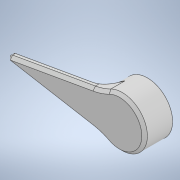
# Autodesk Inventor part: Стрелочка
Saved by Autodesk Inventor 2021.2 (Build 252289000, 289)
## iProperties
Created: 2024-11-30
Part Number: Стрелочка
Material: Типовые
Document SubType Name: Modeling
Designer: Barcock
Density: 1 g/cm^3
Appearance: По умолчанию
Author: Barcock
Autodesk Inventor part; units mm, degrees
ref_plane "YZ Plane" through (0, 0, 0) normal (1, 0, 0) x (0, 1, 0)
ref_plane "XZ Plane" through (0, 0, 0) normal (0, 1, 0) x (-1, 0, 0)
ref_plane "XY Plane" through (0, 0, 0) normal (0, 0, 1) x (1, 0, 0)
sketch "Эскиз1" plane through (0, 0, 0) normal (0, 0, 1) x (1, 0, 0)
  circle A0 centre (0, 0) radius 3.3
  circle A1 centre (0, 0) radius 4.5
  circle A2 centre (0, 0) radius 20 construction
  arc A3 (-19.586824, 0.492404) -> (-19.586824, -0.492404) centre (-19.5, 0) ccw
  line L0 (-19.586824, 0.492404) -> (-4.785745, 3.102233)
  arc A4 (-4.785745, 3.102233) -> (-2.024139, 4.019062) centre (-6.522227, 12.950311) ccw
  line L1 (-19.586824, -0.492404) -> (-4.785745, -3.102233)
  arc A5 (-2.024139, -4.019062) -> (-4.785745, -3.102233) centre (-6.522227, -12.950311) ccw
  dimension "d0" = 6.6
  dimension "d1" = 1.2
  dimension "d2" = 40
  dimension "d3" = 0.5
  dimension "d4" = 20
  dimension "d5" = 10
  constraints: 8 point on circle, 7 tangent, 6 centre point, 4 end point, 3 coincident, 1 equal length, 1 equal radius, 1 horizontal alignment
  measures "d0" diameter of A0
  measures "d1" radial gap between concentric circles of A0 A1
  measures "d2" diameter of A2
  measures "d3" radius of A3
  measures "d4" angle of L1 L0
  measures "d5" radius of A4
extrude "Выдавливание1" add sketch "Эскиз1" against normal blind 1 contours A0 | A1 | A1 A5 L1 A3 L0 A4
extrude "Выдавливание2" add sketch "Эскиз1" against normal blind 1 from surface at -1 contours A0 | A1
extrude "Выдавливание3" add sketch "Эскиз1" against normal blind 3 from surface at -2 contours A1
fillet "Сопряжение1" radius 2 1 edges at (-4.5, 0, -1)
chamfer "Фаска1" distance 0.5 angle 45 7 edges at (-12.1863, 1.7973, 0) (-20, 0, 0) (-12.1863, -1.7973, 0) (-3.3714, -3.4597, 0) (4.5, 0, 0) (-3.3714, 3.4597, 0) (-3.3, 0, -5)
equation "\"d0\" = M4_screw_innerHex_cap_diam"
equation "\"blade_radius\" = 127"
equation "\"bearing_inner\" = 7"
equation "\"bearing_outer\" = 19"
equation "\"bearing_width\" = 6"
equation "\"beam_length\" = 254"
equation "\"motor_height\" = 24"
equation "\"motor_diameter\" = 28"
equation "\"motor_blade_offset\" = 2"
equation "\"M4_screw_innerHex_cap_diam\" = 6.6"
equation "\"M4_screw_innerHex_cap_height\" = 4"
equation "\"M4_nut_lock_width\" = 6.8"
equation "\"M4_nut_lock_height\" = 5"
